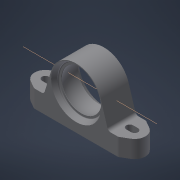
# Autodesk Inventor part: housingSYWK 506 Y-h
Saved by Autodesk Inventor 2022 (Build 260153000, 153)
## iProperties
Category: PARTsolutions
Company: SKF
Part Number: housingSYWK 506 Y-h
Material: Genérico
Catalog Web Link: www.cadenas.de
Description: ayp_001_hc_hh_hy-ayl_001_hp_housing-Plummer block housings for Y-bearings
Vendor: SKF
Document SubType Name: Modeling
Designer: partserver
Manufacturer: SKF
Mass: 127.227 g
Surface Area: 312.414 cm^2
Volume: 127.227 cm^3
Density: 1 g/cm^3
Appearance: PSOLRGB-175-175-175
PSOL_IDENT_0: {$CADENAS_DATA\23d-libs\skf\bearings_units_and_housings\bearing_units\ball_bearing_units\y-units\y-b
PSOL_IDENT_1: earing_plummer_block_units_parts\ayp_001_hc_hh_hy-ayl_001_hp_housing.prj},217 {VTYP=3D},{NB=housingS
PSOL_IDENT_2: YWK 506 Y-h},{LINA=housingSYWK 506 Y-h},{NN=ayp_001_hc_hh_hy-ayl_001_hp_housing},{DATE=20.09.2021 12
PSOL_IDENT_3: :02:20},{GEOMDATE=16.12.2020 09:20:11},{VERSION=},{LINEID=5570},{WBVAR=ENDCOVER},{WBNUMERIC=}  {NB=h
PSOL_IDENT_4: ousingSYWK 506 Y-h},{LINA=housingSYWK 506 Y-h},{KT=DUMMY},{DESIGNATION=SYWK 506 Y},{DESIGN=sywk},{EN
PSOL_IDENT_5: DCOVER=},{ECPN=},{D=62.000},{H1=42.900},{A=40.000},{A1=25.000},{A5=30.500},{H=82.000},{H2=19.000},{J=
PSOL_IDENT_6: 121.000},{L=159.000},{N=21.500},{N1=14.500},{RG=},{R1=MIN},{RA=MIN},{DN=MIN},{SWN=MIN},{GN=},{J6=MIN
PSOL_IDENT_7: },{J7=MIN},{N4=MIN},{MASS=0.210},{G=12.000},{GIN=0.500},{COVER=ECW 206},{PIM=SYWK 506 Y},{LOOKUP=AEC
PSOL_IDENT_8: ALG,DECALG,D1ECALG,D2ECALG},{AEC=33.500},{AECALG=COVER,HEL02,AEC},{DEC=54.100},{DECALG=COVER,HED10,D
PSOL_IDENT_9: EC},{D1EC=64.400},{D1ECALG=COVER,HED13,D1EC},{D2EC=66.000},{D2ECALG=COVER,HED12,D2EC},{PPATH=apb_001
PSOL_IDENT_10: -002_apf_001_app_001_asmtpl.prj},{HIDE=0},{COPYTABLE=apb_001-002_apf_001_app_001_dummy|DUMMY,apb_001
PSOL_IDENT_11: -002_apf_001_app_001_housing|HOUSING,apb_001-002_apf_001_app_001_housing_arc|HOUSING2},{DUMMY=dummy}
PSOL_IDENT_12: ,{HOUSING=housing},{HOUSING2=housing2},{CANGLE=79.258},{ACRL=31.985},{ARCC=5.393},{S=0},{NON=},{DS=0
PSOL_IDENT_13: .000},{NOCUT=},{H3=MIN},{JMAX=128.000},{JMIN=114.000},{A5UP=31.000},{L1=MIN},{H4=MIN},{R2=MIN},{L2=M
PSOL_IDENT_14: IN},{H5=MIN},{L6=MIN},{L7=MIN},{H6=MIN},{L8=MIN},{R3=MIN},{L9=MIN},{ANG=MIN},{L10=MIN},{H7=MIN},{H8=
PSOL_IDENT_15: MIN},{R4=MIN},{R5=MIN},{R6=MIN},{H9=MIN},{ANG1=MIN},{ANG2=MIN},{L11=MIN},{R7=MIN},{L12=MIN},{R8=MIN}
PSOL_IDENT_16: ,{L13=MIN},{H10=MIN},{H11=MIN},{L14=MIN},{R9=MIN},{L15=MIN},{H12=MIN},{L16=MIN},{L17=MIN},{DRAFT=MIN
PSOL_IDENT_17: },{SCALE=MIN}
NB: housingSYWK 506 Y-h
NN: ayp_001_hc_hh_hy-ayl_001_hp_housing
NT: Plummer block housings for Y-bearings
NBSYN: $HOUSING.$DESIGNATION.$ECPN.-h
LINA: housingSYWK 506 Y-h
CATALOG: SKF
DESIGNATION: SYWK 506 Y
DESIGN: sywk
ENDCOVER: w/o End Cover
D: 62
H1: 42.9
A: 40
A1: 25
A5: 30.5
H: 82
H2: 19
J: 121
L: 159
N: 21.5
N1: 14.5
R1: 0
RA: 0
DN: 0
SWN: 0
J6: 0
J7: 0
N4: 0
MASS: 0.21
G: 12
GIN: 0.5
COVER: ECW 206
PIM: SYWK 506 Y
AEC: 33.5
DEC: 54.1
D1EC: 64.4
D2EC: 66
DS: 0
H3: 0
JMAX: 128
JMIN: 114
A5UP: 31
L1: 0
H4: 0
R2: 0
L2: 0
H5: 0
L6: 0
L7: 0
H6: 0
L8: 0
R3: 0
L9: 0
ANG: 0
L10: 0
H7: 0
H8: 0
R4: 0
R5: 0
R6: 0
H9: 0
ANG1: 0
ANG2: 0
L11: 0
R7: 0
L12: 0
R8: 0
L13: 0
H10: 0
H11: 0
L14: 0
R9: 0
L15: 0
H12: 0
L16: 0
L17: 0
DRAFT: 0
SCALE: 0
SUPPLIER: SKF
ARTICLENO: housingSYWK 506 Y-h
BOMINFO: housingSYWK 506 Y-h
CREATOR: CADENAS GmbH
Title: housingSYWK 506 Y-h
Author: Cadenas PARTsolutions
Comments: Plummer block housings for Y-bearings
Autodesk Inventor part; units mm, degrees
ref_plane "YZ Plane" through (0, 0, 0) normal (1, 0, 0) x (0, 1, 0)
ref_plane "XZ Plane" through (0, 0, 0) normal (0, 1, 0) x (-1, 0, 0)
ref_plane "XY Plane" through (0, 0, 0) normal (0, 0, 1) x (1, 0, 0)
sketch "Sketch_1" plane through (0, 0, 0) normal (1, 0, 0) x (0, 1, 0)
  line L0 (0, -20) -> (0, 20)
  line L1 (35.7991, 20) -> (32.5, 14.2857)
  line L2 (32.5, 14.2857) -> (32.5, 13.2857)
  arc A0 (31.5, 12.2857) -> (32.5, 13.2857) centre (31.5, 13.2857) ccw
  line L3 (31.5, 12.2857) -> (28.9616, 12.2857)
  line L4 (28.9616, 12.2857) -> (28.6105, 11.9347)
  arc A1 (28.6105, -11.9347) -> (28.6105, 11.9347) centre (0, 0) ccw
  line L5 (28.6105, -11.9347) -> (28.9616, -12.2857)
  line L6 (28.9616, -12.2857) -> (31.5, -12.2857)
  arc A2 (32.5, -13.2857) -> (31.5, -12.2857) centre (31.5, -13.2857) ccw
  line L7 (32.5, -13.2857) -> (32.5, -14.2857)
  line L8 (32.5, -14.2857) -> (35.7991, -20)
  line L9 (35.7991, -20) -> (119.25, -20)
  line L10 (119.25, -20) -> (119.25, 20)
  line L11 (119.25, 20) -> (35.7991, 20)
  constraints: 24 end point, 6 point on circle, 3 centre point
revolve "Revolution1" add sketch "Sketch_1" angle 360 about axis through (0, 0, -20) along (0, 0, -1)
sketch "Sketch_2" plane through (0, 0, 0) normal (0, 0, 1) x (1, 0, 0)
  circle A0 centre (0, 0) radius 119.25
  line L0 (-79.5, -23.9) -> (-79.5, -42.9)
  line L1 (79.5, -42.9) -> (79.5, -23.9)
  line L2 (79.5, -23.9) -> (49.75, -23.9)
  arc A1 (44.9663, -20.3546) -> (49.75, -23.9) centre (49.75, -18.9) ccw
  line L3 (44.9663, -20.3546) -> (35.4954, 10.7929)
  arc A2 (35.4954, 10.7929) -> (-35.4954, 10.7929) centre (0, 0) ccw
  line L4 (-35.4954, 10.7929) -> (-44.9663, -20.3546)
  arc A3 (-49.75, -23.9) -> (-44.9663, -20.3546) centre (-49.75, -18.9) ccw
  line L5 (-49.75, -23.9) -> (-79.5, -23.9)
  line L6 (79.5, -42.9) -> (79.5, -49)
  line L7 (79.5, -49) -> (-79.5, -49)
  line L8 (-79.5, -49) -> (-79.5, -42.9)
  dimension "d30" = 238.5
  dimension "d31" = 6.1
  constraints: 18 end point, 6 point on circle, 4 centre point, 1 coincident, 1 horizontal, 1 perpendicular, 1 vertical
  measures "d30" diameter of A0
  measures "d31" distance of L1.start L6.end
extrude "Extrusion1" cut sketch "Sketch_2" along normal mid plane 40
sketch "Sketch_3" plane through (0, 0, 0) normal (0, 1, 0) x (-1, 0, 0)
  line L0 (87.45, -22) -> (87.45, 22)
  line L1 (87.45, 22) -> (-87.45, 22)
  line L2 (-87.45, 22) -> (-87.45, -22)
  line L3 (-87.45, -22) -> (87.45, -22)
  arc A0 (71.75, -13.4234) -> (71.75, 13.4234) centre (64, 0) ccw
  line L4 (71.75, 13.4234) -> (61.5192, 19.3301)
  arc A1 (61.5192, 19.3301) -> (59.0192, 20) centre (59.0192, 15) ccw
  line L5 (59.0192, 20) -> (-59.0192, 20)
  arc A2 (-59.0192, 20) -> (-61.5192, 19.3301) centre (-59.0192, 15) ccw
  line L6 (-61.5192, 19.3301) -> (-71.75, 13.4234)
  arc A3 (-71.75, 13.4234) -> (-71.75, -13.4234) centre (-64, 0) ccw
  line L7 (-71.75, -13.4234) -> (-61.5192, -19.3301)
  arc A4 (-61.5192, -19.3301) -> (-59.0192, -20) centre (-59.0192, -15) ccw
  line L8 (-59.0192, -20) -> (59.0192, -20)
  arc A5 (59.0192, -20) -> (61.5192, -19.3301) centre (59.0192, -15) ccw
  line L9 (61.5192, -19.3301) -> (71.75, -13.4234)
  constraints: 20 end point, 12 point on circle, 6 centre point
extrude "Extrusion2" cut sketch "Sketch_3" against normal through all
sketch "Sketch_8" plane through (0, 0, 0) normal (0, 1, 0) x (-1, 0, 0)
  arc A0 (64, -5.5) -> (64, 5.5) centre (64, 0) ccw
  line L0 (64, 5.5) -> (57, 5.5)
  arc A1 (57, 5.5) -> (57, -5.5) centre (57, 0) ccw
  line L1 (57, -5.5) -> (64, -5.5)
  line L2 (0, -28) -> (0, 28) projected
  line L3 (111.3, 0) -> (-111.3, 0) projected
  arc A2 (71.75, -13.4234) -> (71.75, 13.4234) centre (64, 0) ccw projected
  point P0 (69.5, 0)
  point P1 (79.5, 0)
  dimension "d32" = 7
  dimension "d33" = 11
  dimension "d34" = 57
  constraints: 6 point on circle, 4 end point, 4 tangent, 2 centre point, 2 horizontal alignment, 1 horizontal
  measures "d32" distance of A1.centre A0.centre
  measures "d33" distance between parallel lines of L0 L1
  measures "d34" distance from line of L2 A1.centre
extrude "Extrusion4" cut sketch "Sketch_8" against normal through all
sketch "Sketch_10" plane through (0, 0, 0) normal (0, 1, 0) x (-1, 0, 0)
  arc A0 (-57, -5.5) -> (-57, 5.5) centre (-57, 0) ccw
  line L0 (-57, 5.5) -> (-64, 5.5)
  arc A1 (-64, 5.5) -> (-64, -5.5) centre (-64, 0) ccw
  line L1 (-64, -5.5) -> (-57, -5.5)
  line L2 (0, -28) -> (0, 28) projected
  point P0 (57, 0)
  dimension "d35" = 11
  dimension "d36" = 7
  dimension "d37" = 57
  constraints: 4 end point, 4 point on circle, 4 tangent, 2 centre point, 1 horizontal, 1 horizontal alignment
  measures "d35" distance between parallel lines of L0 L1
  measures "d36" distance of A0.centre A1.centre
  measures "d37" distance from line of A0.centre L2
extrude "Extrusion5" cut sketch "Sketch_10" against normal through all
equation "\"d37\" = d34"
body "Solid1"
